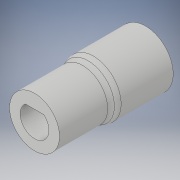
# Autodesk Inventor part: Motor to hex coupler
Saved by Autodesk Inventor 2019 (Build 230136000, 136)
## iProperties
Created: 2022-05-22
Part Number: Motor to hex coupler
Material: Generic
Document SubType Name: Modeling
Designer: Ian
Density: 1 g/cm^3
Appearance: Default
Author: Ian
Autodesk Inventor part; units mm, degrees
ref_plane "YZ Plane" through (0, 0, 0) normal (1, 0, 0) x (0, 1, 0)
ref_plane "XZ Plane" through (0, 0, 0) normal (0, 1, 0) x (-1, 0, 0)
ref_plane "XY Plane" through (0, 0, 0) normal (0, 0, 1) x (1, 0, 0)
sketch "Sketch1" plane through (0, 0, 0) normal (0, 0, 1) x (1, 0, 0)
  arc A0 (-1.6613, 2) -> (1.6613, 2) centre (0, 0) ccw
  line L0 (-1.6613, 2) -> (1.6613, 2)
  circle A1 centre (0, 0) radius 4.5
  dimension "d0" = 5.2
  dimension "d1" = 4.6
  dimension "d2" = 9
  constraints: 2 centre point, 2 coincident, 2 end point, 2 point on circle, 1 horizontal
  measures "d0" diameter of A0
  measures "d2" diameter of A1
extrude "Extrusion1" add sketch "Sketch1" along normal blind 10
sketch "Sketch2" plane through (0, 0, 0) normal (0, 0, -1) x (-1, 0, 0)
  line L0 (1.7898, 3.1) -> (3.5796, 0)
  line L1 (3.5796, 0) -> (1.7898, -3.1)
  line L2 (1.7898, -3.1) -> (-1.7898, -3.1)
  line L3 (-1.7898, -3.1) -> (-3.5796, 0)
  line L4 (-3.5796, 0) -> (-1.7898, 3.1)
  line L5 (-1.7898, 3.1) -> (1.7898, 3.1)
  circle A0 centre (0, 0) radius 5
  dimension "d5" = 6.2
  dimension "d6" = 10
  constraints: 12 end point, 2 coincident, 1 centre point, 1 horizontal, 13 other
  measures "d5" distance between parallel lines of L2 L5
  measures "d6" diameter of A0
extrude "Extrusion2" add sketch "Sketch2" along normal blind 10
fillet "Fillet1" radius 2 2 edges at (-4.5, 0, 0) (5, 0, 0)
body "Solid1"
